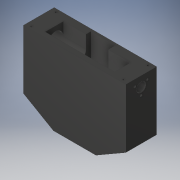
# Autodesk Inventor part: HA01
Saved by Autodesk Inventor 2017 (Build 210142000, 142)
## iProperties
Created: 2018-10-18
Part Number: HA01
Material: ABS Plastic
Document SubType Name: Modeling
Designer: Dell
Density: 1.06 g/cm^3
Appearance: Smooth - Black
Author: Dell
Autodesk Inventor part; units mm, degrees
ref_plane "YZ Plane" through (0, 0, 0) normal (1, 0, 0) x (0, 1, 0)
ref_plane "XZ Plane" through (0, 0, 0) normal (0, 1, 0) x (-1, 0, 0)
ref_plane "XY Plane" through (0, 0, 0) normal (0, 0, 1) x (1, 0, 0)
sketch "Sketch1" plane through (0, 0, 0) normal (0, 0, 1) x (1, 0, 0)
  line L0 (0, -144.3376) -> (-125, -72.1688)
  line L1 (-125, -72.1688) -> (-125, 72.1688)
  line L2 (-125, 72.1688) -> (0, 144.3376) construction
  line L3 (0, 144.3376) -> (125, 72.1688) construction
  line L4 (125, 72.1688) -> (125, -72.1688)
  line L5 (125, -72.1688) -> (0, -144.3376)
  line L6 (125, 72.1688) -> (-125, 72.1688)
  line L7 (125, 72.1688) -> (-125, 72.1688)
  line L8 (-125, 72.1688) -> (-125, 144.3376)
  line L9 (-125, 144.3376) -> (125, 144.3376)
  line L10 (125, 144.3376) -> (125, 72.1688)
  point P0 (0, 0)
  point P1 (0, 0)
  dimension "d0" = 250
  constraints: 22 end point, 2 horizontal, 2 parallel, 2 vertical alignment, 1 coincident, 1 midpoint, 1 perpendicular, 13 other
  measures "d0" distance between parallel lines of L4 L1
extrude "Extrusion1" add sketch "Sketch1" along normal blind 75 contours L0 L1 L6 L4 L5
sketch "Sketch2" plane through (-125, 72.1688, 0) normal (0, 1, 0) x (1, 0, 0)
  line L0 (200, -55) -> (50, -55)
  line L1 (50, -55) -> (50, -20)
  line L2 (50, -20) -> (200, -20)
  line L3 (200, -20) -> (200, -55)
  line L4 (0, 0) -> (0, -75) projected
  line L5 (0, 0) -> (250, 0) projected
  point P0 (125, -20)
  point P1 (50, -37.5)
  point P2 (125, 0)
  point P3 (0, -37.5)
  dimension "d3" = 150
  dimension "d4" = 35
  constraints: 8 end point, 4 midpoint, 2 parallel, 1 horizontal, 1 horizontal alignment, 1 perpendicular, 1 vertical alignment
  measures "d3" distance of L0.start L0.end
  measures "d4" distance of L0.end L1.end
extrude "Extrusion2" cut sketch "Sketch2" against normal through all
sketch "Sketch3" plane through (0, 0, 75) normal (0, 0, 1) x (1, 0, 0)
  line L0 (125, -114.3376) -> (-125, -114.3376)
  line L1 (-125, -114.3376) -> (-125, -144.3376)
  line L2 (-125, -144.3376) -> (125, -144.3376)
  line L3 (125, -144.3376) -> (125, -114.3376)
  point P0 (0, 0)
  point P1 (0, -144.3376)
  point P2 (0, -114.3376)
  point P3 (125, -72.1688)
  dimension "d7" = 30
  constraints: 8 end point, 2 parallel, 2 vertical alignment, 1 horizontal, 1 horizontal alignment, 1 midpoint, 1 perpendicular
  measures "d7" distance of L2.end L0.start
extrude "Extrusion3" cut sketch "Sketch3" against normal through all
sketch "Sketch4" plane through (125, -72.1688, 0) normal (1, 0, 0) x (0, 0, -1)
  circle A0 centre (-37.5, 119.3376) radius 3
  line L0 (0, 144.3376) -> (-75, 144.3376) projected
  point P0 (-37.5, 144.3376)
  dimension "d14" = 6
  dimension "d15" = 25
  constraints: 1 centre point, 1 midpoint, 1 vertical alignment
  measures "d14" diameter of A0
  measures "d15" distance from line of L0 A0.centre
extrude "Extrusion4" cut sketch "Sketch4" against normal through all
sketch "Sketch5" plane through (-125, -72.1688, 0) normal (-1, 0, 0) x (0, 0, 1)
  circle A0 centre (37.5, 119.3376) radius 3 projected
  circle A1 centre (37.5, 112.3376) radius 1.5
  circle A2 centre (53, 112.3376) radius 1.5
  circle A3 centre (45.25, 125.761) radius 1.5
  circle A4 centre (29.75, 125.761) radius 1.5
  circle A5 centre (22, 112.3376) radius 1.5
  circle A6 centre (29.75, 98.9142) radius 1.5
  circle A7 centre (45.25, 98.9142) radius 1.5
  circle A8 centre (37.5, 119.3376) radius 6
  point P0 (0, 72.1688)
  dimension "d16" = 3
  dimension "d17" = 3
  dimension "d18" = 7
  dimension "d19" = 15.5
  dimension "d22" = 360
  dimension "d26" = 12
  constraints: 8 centre point, 1 coincident, 1 horizontal alignment, 1 vertical alignment, 13 other
  measures "d16" diameter of A1
  measures "d17" diameter of A2
  measures "d18" distance of A0.centre A1.centre
  measures "d19" distance of A1.centre A2.centre
  measures "d26" diameter of A8
extrude "Extrusion5" cut sketch "Sketch5" against normal blind 75 contours A0 | A8 A1 | A1 A8 | A2 | A3 | A4 | A5 | A6 | A7 picked at (37.446, 113.508) picked at (36.0874, 114.6648)
sketch "Sketch6" plane through (-75, 72.1688, 55) normal (1, 0, 0) x (0, 0, -1)
  circle A0 centre (17.5, -32) radius 20
  circle A1 centre (33, -32) radius 1.5 projected
  circle A2 centre (17.5, -25) radius 6 projected
  point P0 (55, -72.1688)
  dimension "d27" = 40
  constraints: 1 centre point, 1 horizontal alignment, 1 vertical alignment
  measures "d27" diameter of A0
extrude "Extrusion6" cut sketch "Sketch6" along normal blind 150 and the other way blind 45 contours A0 | A1 | A2
sketch "Sketch7" plane through (-125, 72.1688, 0) normal (0, 1, 0) x (1, 0, 0)
  line L0 (50, -12.5) -> (200, -12.5)
  line L1 (200, -12.5) -> (200, -62.5)
  line L2 (200, -62.5) -> (50, -62.5)
  line L3 (50, -62.5) -> (50, -12.5)
  line L4 (50, -55) -> (50, -20) projected
  line L5 (200, -20) -> (200, -55) projected
  point P0 (125, 0)
  point P1 (50, -37.5)
  dimension "d32" = 50
  constraints: 8 end point, 2 midpoint, 2 parallel, 2 vertical alignment, 1 horizontal, 1 perpendicular
  measures "d32" distance of L2.end L0.start
extrude "Extrusion7" cut sketch "Sketch7" against normal blind 50
sketch "Sketch8" plane through (-125, 72.1688, 0) normal (0, 1, 0) x (1, 0, 0)
  line L0 (12.5, -7.5) -> (237.5, -7.5) construction
  line L1 (237.5, -7.5) -> (237.5, -67.5) construction
  line L2 (237.5, -67.5) -> (12.5, -67.5) construction
  line L3 (12.5, -67.5) -> (12.5, -7.5) construction
  line L4 (50, -62.5) -> (50, -12.5) construction
  line L5 (50, -12.5) -> (200, -12.5) construction
  circle A0 centre (12.5, -7.5) radius 2.5
  circle A1 centre (12.5, -67.5) radius 2.5
  circle A2 centre (237.5, -67.5) radius 2.5
  circle A3 centre (237.5, -7.5) radius 2.5
  point P0 (125, 0)
  point P1 (125, -12.5)
  point P2 (125, -12.5)
  point P3 (125, -7.5)
  point P4 (50, -37.5)
  point P5 (12.5, -37.5)
  dimension "d35" = 225
  dimension "d36" = 60
  dimension "d37" = 5
  dimension "d38" = 5
  dimension "d39" = 5
  dimension "d40" = 5
  constraints: 8 end point, 5 midpoint, 4 centre point, 4 coincident, 2 parallel, 1 horizontal, 1 horizontal alignment, 1 perpendicular, 1 vertical alignment
  measures "d35" distance of L0.start L0.end
  measures "d36" distance of L2.end L0.start
  measures "d37" diameter of A0
  measures "d38" diameter of A1
  measures "d39" diameter of A2
  measures "d40" diameter of A3
extrude "Extrusion8" cut sketch "Sketch8" against normal blind 50
sketch "Sketch9" plane through (-125, -72.1688, 0) normal (-1, 0, 0) x (0, 0, 1)
  circle A0 centre (22, 112.3376) radius 1.5 construction
  circle A1 centre (37.5, 119.3376) radius 3 construction
  line L0 (22, 112.3376) -> (37.5, 112.3376) construction
  circle A2 centre (37.5, 119.3376) radius 6 construction
  line L1 (37.5, 112.3376) -> (37.5, 119.3376) construction
  circle A3 centre (22, 112.3376) radius 4
  circle A4 centre (29.75, 98.9142) radius 4
  circle A5 centre (45.25, 98.9142) radius 4
  circle A6 centre (53, 112.3376) radius 4
  circle A7 centre (45.25, 125.761) radius 4
  circle A8 centre (29.75, 125.761) radius 4
  point P0 (0, 72.1688)
  dimension "d43" = 8
  dimension "d46" = 360
  constraints: 6 centre point, 4 end point, 1 coincident, 1 horizontal, 1 perpendicular, 13 other
  measures "d43" diameter of A3
extrude "Extrusion9" cut sketch "Sketch9" against normal blind 3
sketch "Sketch10" plane through (-120, 40.1688, 37.5) normal (1, 0, 0) x (0, 0, -1)
  circle A0 centre (0, 7) radius 6 projected
  circle A1 centre (7.75, -13.4234) radius 1.5 projected
  circle A2 centre (7.75, 13.4234) radius 1.5 projected
  circle A3 centre (-15.5, 0) radius 1.5 projected
  circle A4 centre (-7.75, 13.4234) radius 1.5 projected
  circle A5 centre (15.5, 0) radius 1.5 projected
  circle A6 centre (-7.75, -13.4234) radius 1.5 projected
  circle A7 centre (0, 0) radius 20 projected
  point P0 (37.5, -40.1688)
extrude "Extrusion10" add sketch "Sketch10" along normal blind 5
sketch "Sketch11" plane through (-125, 72.1688, 0) normal (0, 1, 0) x (1, 0, 0)
  line L0 (155, -62.5) -> (95, -62.5)
  line L1 (95, -62.5) -> (95, -5)
  line L2 (95, -5) -> (155, -5)
  line L3 (155, -5) -> (155, -62.5)
  line L4 (210, -62.5) -> (40, -62.5)
  line L5 (40, -62.5) -> (40, -27.5)
  line L6 (210, -27.5) -> (210, -62.5)
  line L7 (210, -27.5) -> (40, -27.5)
  line L8 (50, -12.5) -> (200, -12.5) projected
  line L9 (200, -62.5) -> (50, -62.5) projected
  point P0 (125, 0)
  point P1 (125, -5)
  point P2 (125, -62.5)
  point P3 (125, -62.5)
  point P4 (125, -12.5)
  dimension "d52" = 60
  dimension "d56" = 170
  dimension "d57" = 35
  dimension "d62" = 7.5
  constraints: 16 end point, 6 midpoint, 3 horizontal, 3 parallel, 2 perpendicular, 1 vertical alignment
  measures "d52" distance of L1.end L2.end
  measures "d56" distance of L4.start L4.end
  measures "d57" distance between parallel lines of L4 L7
  measures "d62" distance between parallel lines of L8 L2
extrude "Extrusion11" cut sketch "Sketch11" against normal blind 165
sketch "Sketch12" plane through (0, 0, 0) normal (0, 0, -1) x (-1, 0, 0)
  line L0 (75, 72.1688) -> (30, 72.1688) projected
  line L1 (75, 72.1688) -> (75, 22.1688) projected
  line L2 (75, 22.1688) -> (30, 22.1688) projected
  line L3 (-30, 22.1688) -> (-75, 22.1688) projected
  line L4 (-75, 72.1688) -> (-75, 22.1688) projected
  circle A0 centre (0, -67.8312) radius 4
  line L5 (-30, 72.1688) -> (-30, 22.1688) projected
  line L6 (-30, 72.1688) -> (-75, 72.1688) projected
  line L7 (30, 22.1688) -> (30, 72.1688) projected
  line L8 (-30, -92.8312) -> (30, -92.8312) projected
  point P0 (0, 0)
  point P1 (0, -92.8312)
  dimension "d58" = 8
  dimension "d65" = 25
  constraints: 1 centre point, 1 midpoint, 1 vertical alignment
  measures "d58" diameter of A0
  measures "d65" distance from line of A0.centre L8
extrude "Extrusion12" cut sketch "Sketch12" against normal blind 25 contours A0
sketch "Sketch13" plane through (-51.9615, -114.3376, 20) normal (0, 0, 1) x (1, 0, 0)
  line L0 (21.9615, 21.5064) -> (21.9615, 136.5064) projected
  line L1 (21.9615, 136.5064) -> (-23.0385, 136.5064) projected
  line L2 (-23.0385, 136.5064) -> (-23.0385, 13.3013) projected
  line L3 (0, 0) -> (-23.0385, 13.3013) projected
  line L4 (0, 0) -> (103.923, 0) projected
  line L5 (126.9615, 13.3013) -> (103.923, 0) projected
  line L6 (126.9615, 136.5064) -> (126.9615, 13.3013) projected
  line L7 (126.9615, 136.5064) -> (81.9615, 136.5064) projected
  line L8 (81.9615, 136.5064) -> (81.9615, 21.5064) projected
  line L9 (81.9615, 21.5064) -> (21.9615, 21.5064) projected
  point P0 (51.9615, 114.3376)
extrude "Extrusion13" add sketch "Sketch13" along normal blind 3
sketch "Sketch15" plane through (-75, 22.1688, 12.5) normal (1, 0, 0) x (0, 0, -1)
  line L0 (-10.5, 0) -> (0, 0) projected
  line L1 (0, 50) -> (0, 0) projected
  line L2 (-15, 50) -> (0, 50) projected
  line L3 (-15, 50) -> (-15, 35.3205) projected
  arc A0 (-15, 0.6795) -> (-15, 35.3205) centre (-25, 18) ccw projected
  line L4 (-15, 0.6795) -> (-15, -115) projected
  line L5 (-15, -115) -> (-42.5, -115) projected
  line L6 (-42.5, -115) -> (-42.5, -123.2051) projected
  line L7 (-10.5, -123.2051) -> (-42.5, -123.2051) projected
  line L8 (-10.5, -123.2051) -> (-10.5, 0) projected
  line L9 (-10.5, 0) -> (-10.5, 4.225)
  line L10 (-10.5, 31.775) -> (-10.5, 50)
  arc A1 (-10.5, 4.225) -> (-10.5, 31.775) centre (-25, 18) ccw
  point P0 (12.5, -22.1688)
  constraints: 4 end point, 4 point on circle, 3 point on line, 1 centre point, 1 concentric, 1 vertical
extrude "Extrusion14" add sketch "Sketch15" along normal blind 45 contours L9 A0 L10 L2 L1 L0
sketch "Sketch16" plane through (75, 22.1688, 12.5) normal (-1, 0, 0) x (0, 0, 1)
  line L0 (0, 0) -> (10.5, 0) projected
  line L1 (10.5, 0) -> (10.5, -123.2051) projected
  line L2 (42.5, -123.2051) -> (10.5, -123.2051) projected
  line L3 (42.5, -115) -> (42.5, -123.2051) projected
  line L4 (42.5, -115) -> (15, -115) projected
  line L5 (15, -115) -> (15, 50) projected
  line L6 (0, 50) -> (15, 50) projected
  line L7 (0, 50) -> (0, 0) projected
  line L8 (10.5, 0) -> (10.5, -123.2051) projected
  line L9 (10.5, 0) -> (10.5, 50)
  line L10 (-12.5, 50) -> (62.5, 50) projected
  line L11 (10.5, 50) -> (0, 50)
  line L12 (-2.5, 50) -> (-2.5, 0) projected
  point P0 (-12.5, -22.1688)
  constraints: 4 end point, 1 perpendicular, 1 point on line, 1 vertical
extrude "Extrusion15" add sketch "Sketch16" along normal blind 45 contours L7 L6 L9 L0
sketch "Sketch17" plane through (-125, -92.8312, 0) normal (0, 1, 0) x (1, 0, 0)
  line L0 (200, -27.5) -> (210, -27.5) projected
  line L1 (200, -23) -> (200, -27.5) projected
  line L2 (50, -27.5) -> (50, -23) projected
  line L3 (40, -27.5) -> (50, -27.5) projected
  line L4 (176.9615, -23) -> (200, -23) projected
  line L5 (200, -23) -> (210, -23)
  line L6 (210, -23) -> (210, -27.5)
  line L7 (210, -27.5) -> (200, -27.5)
  line L8 (200, -27.5) -> (200, -23)
  line L9 (50, -23) -> (73.0385, -23) projected
  line L10 (50, -23) -> (40, -23)
  line L11 (40, -23) -> (40, -27.5)
  line L12 (40, -27.5) -> (50, -27.5)
  line L13 (50, -27.5) -> (50, -23)
  point P0 (125, 0)
  constraints: 16 end point, 4 parallel, 2 horizontal, 2 perpendicular
extrude "Extrusion16" cut sketch "Sketch17" along normal through all
sketch "Sketch18" plane through (-85, -92.8312, 62.5) normal (1, 0, 0) x (0, 0, -1)
  arc A0 (39.5, 119.225) -> (39.5, 146.775) centre (25, 133) ccw projected
  line L0 (57.5, 165) -> (39.5, 165) projected
  circle A1 centre (25, 133) radius 20 projected
  line L1 (45, 133) -> (39.5, 133)
  line L2 (39.5, 133) -> (39.5, 165)
  line L3 (39.5, 165) -> (45, 165)
  line L4 (45, 165) -> (45, 133)
  point P0 (62.5, 92.8312)
  constraints: 8 end point, 2 parallel, 2 point on circle, 1 horizontal, 1 perpendicular
extrude "Extrusion17" cut sketch "Sketch18" along normal blind 55 contours L1 L2 A0 | A0 L2 L0 L4
sketch "Sketch20" plane through (85, -92.8312, 62.5) normal (-1, 0, 0) x (0, 0, 1)
  circle A0 centre (-25, 140) radius 3 projected
  circle A1 centre (-25, 140) radius 11.5
  point P0 (-62.5, 92.8312)
  dimension "d74" = 23
  constraints: 1 centre point, 1 coincident
  measures "d74" diameter of A1
extrude "Extrusion18" cut sketch "Sketch20" against normal through all
sketch "Sketch21" plane through (125, -72.1688, 0) normal (1, 0, 0) x (0, 0, -1)
  circle A0 centre (-37.5, 119.3376) radius 11.5 projected
  circle A1 centre (-37.5, 101.8376) radius 2.5
  circle A2 centre (-22.3446, 128.0876) radius 2.5
  circle A3 centre (-52.6554, 128.0876) radius 2.5
  point P0 (0, 72.1688)
  dimension "d77" = 17.5
  dimension "d78" = 5
  dimension "d81" = 360
  constraints: 3 centre point, 1 vertical alignment, 7 other
  measures "d77" distance of A0.centre A1.centre
  measures "d78" diameter of A1
extrude "Extrusion19" cut sketch "Sketch21" against normal blind 35 contours A1 | A2 | A3
sketch "Sketch22" plane through (0, 0, 0) normal (0, 0, -1) x (-1, 0, 0)
  circle A0 centre (0, -67.8312) radius 4 projected
  circle A1 centre (0, -67.8312) radius 10
  point P0 (0, 0)
  dimension "d85" = 20
  constraints: 1 centre point, 1 coincident
  measures "d85" diameter of A1
extrude "Extrusion20" cut sketch "Sketch22" against normal blind 2
body "Solid1"
